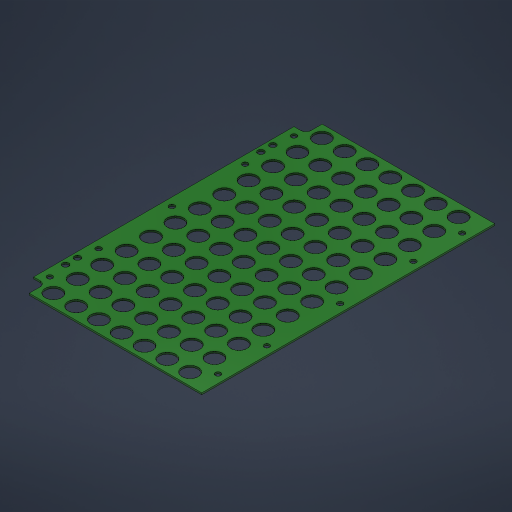
# Autodesk Inventor part: PCB
Saved by Autodesk Inventor 2023.5 (Build 275446000, 446)
## iProperties
Created: 2025-03-26
Part Number: PCB
Material: PC/ABS-Kunststoff
Document SubType Name: Modeling
Designer: David Lill
Density: 0.357273 g/cm^3
Appearance: Glatt - Waldgrün
Author: David Lill
Autodesk Inventor part; units mm, degrees
ref_plane "YZ Plane" through (0, 0, 0) normal (1, 0, 0) x (0, 1, 0)
ref_plane "XZ Plane" through (0, 0, 0) normal (0, 1, 0) x (-1, 0, 0)
ref_plane "XY Plane" through (0, 0, 0) normal (0, 0, 1) x (1, 0, 0)
sketch "Skizze1" plane through (0, 0, 0) normal (0, 0, 1) x (1, 0, 0)
  line L0 (-159, 270) -> (-159, 260)
  arc A0 (-164, 255) -> (-159, 260) centre (-164, 260) ccw
  line L1 (-164, 255) -> (-170, 255)
  line L2 (-170, 255) -> (-170, 15)
  line L3 (-170, 15) -> (-164, 15)
  arc A1 (-159, 10) -> (-164, 15) centre (-164, 10) ccw
  line L4 (-159, 10) -> (-159, 0)
  line L5 (-159, 0) -> (0, 0)
  line L6 (0, 0) -> (0, 270)
  line L7 (0, 270) -> (-159, 270)
  circle A2 centre (-162.5, 202.5) radius 2.5
  circle A3 centre (-7.5, 135) radius 2.5
  circle A4 centre (-162.5, 135) radius 2.5
  circle A5 centre (-162.5, 22.5) radius 2.5
  circle A6 centre (-7.5, 67.5) radius 2.5
  circle A7 centre (-7.5, 202.5) radius 2.5
  circle A8 centre (-162.5, 247.5) radius 2.5
  circle A9 centre (-7.5, 22.5) radius 2.5
  circle A10 centre (-7.5, 247.5) radius 2.5
  circle A11 centre (-162.5, 67.5) radius 2.5
  circle A12 centre (-148, 258.75) radius 7.5
  circle A13 centre (-148, 213.75) radius 7.5
  circle A14 centre (-148, 168.75) radius 7.5
  circle A15 centre (-148, 123.75) radius 7.5
  circle A16 centre (-148, 78.75) radius 7.5
  circle A17 centre (-148, 33.75) radius 7.5
  circle A18 centre (-148, 11.25) radius 7.5
  circle A19 centre (-148, 56.25) radius 7.5
  circle A20 centre (-148, 101.25) radius 7.5
  circle A21 centre (-148, 146.25) radius 7.5
  circle A22 centre (-148, 191.25) radius 7.5
  circle A23 centre (-148, 236.25) radius 7.5
  circle A24 centre (-127, 191.25) radius 7.5
  circle A25 centre (-127, 146.25) radius 7.5
  circle A26 centre (-127, 101.25) radius 7.5
  circle A27 centre (-127, 56.25) radius 7.5
  circle A28 centre (-127, 11.25) radius 7.5
  circle A29 centre (-127, 33.75) radius 7.5
  circle A30 centre (-127, 78.75) radius 7.5
  circle A31 centre (-127, 123.75) radius 7.5
  circle A32 centre (-127, 168.75) radius 7.5
  circle A33 centre (-127, 213.75) radius 7.5
  circle A34 centre (-127, 258.75) radius 7.5
  circle A35 centre (-127, 236.25) radius 7.5
  circle A36 centre (-106, 191.25) radius 7.5
  circle A37 centre (-106, 146.25) radius 7.5
  circle A38 centre (-106, 101.25) radius 7.5
  circle A39 centre (-106, 56.25) radius 7.5
  circle A40 centre (-106, 11.25) radius 7.5
  circle A41 centre (-106, 33.75) radius 7.5
  circle A42 centre (-106, 78.75) radius 7.5
  circle A43 centre (-106, 123.75) radius 7.5
  circle A44 centre (-106, 168.75) radius 7.5
  circle A45 centre (-106, 213.75) radius 7.5
  circle A46 centre (-106, 258.75) radius 7.5
  circle A47 centre (-106, 236.25) radius 7.5
  circle A48 centre (-85, 191.25) radius 7.5
  circle A49 centre (-85, 146.25) radius 7.5
  circle A50 centre (-85, 101.25) radius 7.5
  circle A51 centre (-85, 56.25) radius 7.5
  circle A52 centre (-85, 11.25) radius 7.5
  circle A53 centre (-85, 33.75) radius 7.5
  circle A54 centre (-85, 78.75) radius 7.5
  circle A55 centre (-85, 123.75) radius 7.5
  circle A56 centre (-85, 168.75) radius 7.5
  circle A57 centre (-85, 213.75) radius 7.5
  circle A58 centre (-85, 258.75) radius 7.5
  circle A59 centre (-85, 236.25) radius 7.5
  circle A60 centre (-64, 191.25) radius 7.5
  circle A61 centre (-64, 146.25) radius 7.5
  circle A62 centre (-64, 101.25) radius 7.5
  circle A63 centre (-64, 56.25) radius 7.5
  circle A64 centre (-64, 11.25) radius 7.5
  circle A65 centre (-64, 33.75) radius 7.5
  circle A66 centre (-64, 78.75) radius 7.5
  circle A67 centre (-64, 123.75) radius 7.5
  circle A68 centre (-64, 168.75) radius 7.5
  circle A69 centre (-64, 213.75) radius 7.5
  circle A70 centre (-64, 258.75) radius 7.5
  circle A71 centre (-64, 236.25) radius 7.5
  circle A72 centre (-43, 191.25) radius 7.5
  circle A73 centre (-43, 146.25) radius 7.5
  circle A74 centre (-43, 101.25) radius 7.5
  circle A75 centre (-43, 56.25) radius 7.5
  circle A76 centre (-43, 11.25) radius 7.5
  circle A77 centre (-43, 33.75) radius 7.5
  circle A78 centre (-43, 78.75) radius 7.5
  circle A79 centre (-43, 123.75) radius 7.5
  circle A80 centre (-43, 168.75) radius 7.5
  circle A81 centre (-43, 213.75) radius 7.5
  circle A82 centre (-43, 258.75) radius 7.5
  circle A83 centre (-43, 236.25) radius 7.5
  circle A84 centre (-22, 191.25) radius 7.5
  circle A85 centre (-22, 146.25) radius 7.5
  circle A86 centre (-22, 101.25) radius 7.5
  circle A87 centre (-22, 56.25) radius 7.5
  circle A88 centre (-22, 11.25) radius 7.5
  circle A89 centre (-22, 33.75) radius 7.5
  circle A90 centre (-22, 78.75) radius 7.5
  circle A91 centre (-22, 123.75) radius 7.5
  circle A92 centre (-22, 168.75) radius 7.5
  circle A93 centre (-22, 213.75) radius 7.5
  circle A94 centre (-22, 258.75) radius 7.5
  circle A95 centre (-22, 236.25) radius 7.5
  point P0 (-159, 0)
  constraints: 96 centre point, 16 end point, 4 point on circle
extrude "Extrusion1" add sketch "Skizze1" along normal blind 1.6
sketch "Skizze2" plane through (0, 0, 1.6) normal (0, 0, 1) x (1, 0, 0)
  circle A0 centre (-165, 230.5) radius 2.85
  circle A1 centre (-165, 219.5) radius 2.85
  line L0 (-170, 255) -> (-170, 15) projected
  line L1 (0, 270) -> (-159, 270) projected
  line L2 (-170, 135) -> (0, 135)
  circle A2 centre (-165, 39.5) radius 2.85
  circle A3 centre (-165, 50.5) radius 2.85
  point P0 (0, 0)
  dimension "d2" = 5.7
  dimension "d3" = 11
  dimension "d4" = 5
  dimension "d5" = 39.5
  constraints: 4 centre point, 2 end point, 2 symmetric about line, 1 equal radius, 1 horizontal, 1 midpoint, 1 vertical alignment, 2 other
  measures "d2" diameter of A0
  measures "d3" distance of A1.centre A0.centre
  measures "d4" distance from line of L0 A0.centre
  measures "d5" distance from line of L1 A0.centre
extrude "Extrusion2" cut sketch "Skizze2" against normal through all
